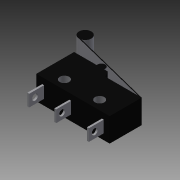
# Autodesk Inventor part: endstopLever
Saved by Autodesk Inventor 2013 (Build 170138000, 138)
## iProperties
Created: 2015-01-14
Part Number: endstopLever
Material: Generic
Document SubType Name: Modeling
Designer: dzban
Density: 1 g/cm^3
Author: dzban
Autodesk Inventor part; units mm, degrees
ref_plane "YZ Plane" through (0, 0, 0) normal (1, 0, 0) x (0, 1, 0)
ref_plane "XZ Plane" through (0, 0, 0) normal (0, 1, 0) x (-1, 0, 0)
ref_plane "XY Plane" through (0, 0, 0) normal (0, 0, 1) x (1, 0, 0)
sketch "Sketch1" plane through (0, 0, 0) normal (0, 0, 1) x (1, 0, 0)
  line L0 (0, 0) -> (0, 10.2)
  line L1 (0, 10.2) -> (9.1, 10.2)
  line L2 (9.1, 10.2) -> (9.99, 8.6487)
  line L3 (9.99, 8.6487) -> (19.8, 8.6487)
  line L4 (19.8, 8.6487) -> (19.8, 0)
  line L5 (19.8, 0) -> (0, 0)
  circle A0 centre (5.1, 2.5) radius 1.25
  circle A1 centre (14.6, 2.5) radius 1.25
  arc A2 (8.1, 10.5) -> (6.1001, 10.4874) centre (7.1, 10.5) ccw
  line L6 (8.1, 10.5) -> (8.1, 10.2)
  line L7 (6.1001, 10.5) -> (6.1001, 10.2)
  dimension "d0" = 9.1
  dimension "d1" = 10.2
  dimension "d2" = 19.8
  dimension "d3" = 2.5
  dimension "d4" = 5.1
  dimension "d5" = 2.5
  dimension "d6" = 9.5
  dimension "d7" = 2.5
  dimension "d8" = 2.5
  dimension "d9" = 2
  dimension "d10" = 7.5
  dimension "d11" = 10.5
  constraints: 16 end point, 5 parallel, 4 point on line, 3 centre point, 2 point on circle, 1 tangent
  measures "d0" distance of L1.start L2.start
  measures "d1" distance between parallel lines of L1 L5
  measures "d2" distance between parallel lines of L0 L4
  measures "d3" diameter of A0
  measures "d4" distance from line of L0 A0.centre
  measures "d5" diameter of A1
  measures "d6" distance of A1.centre A0.centre
  measures "d7" distance from line of L5 A1.centre
  measures "d8" distance from line of L5 A0.centre
  measures "d9" diameter of A2
  measures "d10" horizontal distance of A2.centre A1.centre
  measures "d11" distance from line of A2.centre L5
extrude "Extrusion1" add sketch "Sketch1" along normal blind 6.4
sketch "Sketch3" plane through (0, 0, 0) normal (0, -1, 0) x (1, 0, 0)
  line L0 (8.9, 1.6) -> (8.9, 4.8)
  line L1 (8.9, 4.8) -> (9.4, 4.8)
  line L2 (9.4, 4.8) -> (9.4, 1.6)
  line L3 (9.4, 1.6) -> (8.9, 1.6)
  line L4 (17.7, 1.6) -> (17.7, 4.8)
  line L5 (17.7, 4.8) -> (18.2, 4.8)
  line L6 (18.2, 4.8) -> (18.2, 1.6)
  line L7 (18.2, 1.6) -> (17.7, 1.6)
  line L8 (1.6, 1.6) -> (1.6, 4.8)
  line L9 (1.6, 4.8) -> (2.1, 4.8)
  line L10 (2.1, 4.8) -> (2.1, 1.6)
  line L11 (2.1, 1.6) -> (1.6, 1.6)
  constraints: 24 end point
extrude "Extrusion3" add sketch "Sketch3" along normal blind 4
sketch "Sketch4" plane through (18.2, 0, 4.8) normal (1, 0, 0) x (0, 0, -1)
  circle A0 centre (1.6, -2.4215) radius 0.8
  point P0 (4.8, 0)
  dimension "d24" = 1.6
  constraints: 1 centre point
  measures "d24" diameter of A0
extrude "Extrusion4" cut sketch "Sketch4" against normal blind 22
sketch "Sketch5" plane through (0, 0, 6.4) normal (0, 0, 1) x (1, 0, 0)
  line L0 (19.8, 8.6487) -> (9.99, 8.6487) projected
  line L1 (18.8606, 8.6487) -> (-2.9473, 14.1382)
  line L2 (-2.9473, 14.1382) -> (-2.4872, 14.2588)
  line L3 (-2.4872, 14.2588) -> (19.8, 8.6487)
  circle A0 centre (-2.4872, 15.6717) radius 1.6664
  constraints: 6 end point, 1 centre point, 1 parallel, 1 point on line
extrude "Extrusion5" add sketch "Sketch5" against normal blind 6.4
sketch "Sketch2" plane through (0, 0, 6.4) normal (0, 0, 1) x (1, 0, 0)
  line L0 (1.6916, 0) -> (2.1916, 0)
  line L1 (2.1916, 0) -> (2.1916, -4)
  line L2 (2.1916, -4) -> (1.6916, -4)
  line L3 (1.6916, -4) -> (1.6916, 0)
  line L4 (10.4916, 0) -> (10.9916, 0)
  line L5 (10.9916, 0) -> (10.9916, -4)
  line L6 (10.9916, -4) -> (10.4916, -4)
  line L7 (10.4916, -4) -> (10.4916, 0)
  line L8 (17.7916, 0) -> (18.2916, 0)
  line L9 (18.2916, 0) -> (18.2916, -4)
  line L10 (18.2916, -4) -> (17.7916, -4)
  line L11 (17.7916, -4) -> (17.7916, 0)
  point P0 (0, 0)
  point P1 (-19.8, 0)
  dimension "d14" = 0.5
  dimension "d15" = 4
  dimension "d16" = 0.5
  dimension "d17" = 0.5
  dimension "d18" = 8.3
  dimension "d19" = 6.8
  constraints: 24 end point, 6 parallel, 3 horizontal, 3 perpendicular
  measures "d14" distance of L1.end L3.start
  measures "d15" distance of L1.start L1.end
  measures "d16" distance of L5.end L6.end
  measures "d17" distance of L9.end L10.end
  measures "d18" distance between parallel lines of L7 L1
  measures "d19" distance between parallel lines of L11 L5
body "Solid1"
